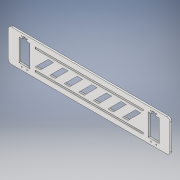
# Autodesk Inventor part: Cuerpo - LateralPrueba
Saved by Autodesk Inventor 2019 (Build 230136000, 136)
## iProperties
Created: 2020-02-14
Part Number: Cuerpo - LateralPrueba
Material: ABS Plastic
Document SubType Name: Modeling
Designer: Mafer1
Density: 1.06 g/cm^3
Appearance: Smooth - White
Mass: 36.6909 g
Surface Area: 287.559 cm^2
Volume: 34.614 cm^3
base_servo: 20.000 mm
altura_servo: 40.000 mm
agujero_servo: 2.000 mm
distancia_agujero_servo: 4.750 mm
soporte: 60.000 mm
largo_base: 200.000 mm
d199: 2.000 mm
d201: 20.000 mm
Author: Mafer1
Autodesk Inventor part; units mm, degrees
ref_plane "YZ Plane" through (0, 0, 0) normal (1, 0, 0) x (0, 1, 0)
ref_plane "XZ Plane" through (0, 0, 0) normal (0, 1, 0) x (-1, 0, 0)
ref_plane "XY Plane" through (0, 0, 0) normal (0, 0, 1) x (1, 0, 0)
sketch "Sketch7" plane through (0, 0, 0) normal (0, 0, 1) x (1, 0, 0)
  line L0 (0, 0) -> (300, 0)
  line L1 (300, 0) -> (300, 60)
  line L2 (300, 60) -> (0, 60)
  line L3 (0, 60) -> (0, 0)
  line L4 (50, 13) -> (250, 13)
  line L5 (250, 13) -> (250, 10)
  line L6 (250, 10) -> (50, 10)
  line L7 (50, 10) -> (50, 13)
  line L8 (150, 13) -> (150, 10) construction
  line L9 (20, 50.8) -> (40.3, 50.8)
  line L10 (40.3, 50.8) -> (40.3, 10)
  line L11 (40.3, 10) -> (20, 10)
  line L12 (20, 10) -> (20, 50.8)
  line L13 (259.7, 50.8) -> (280, 50.8)
  line L14 (280, 50.8) -> (280, 10)
  line L15 (280, 10) -> (259.7, 10)
  line L16 (259.7, 10) -> (259.7, 50.8)
  line L17 (50, 47) -> (250, 47)
  line L18 (250, 47) -> (250, 50)
  line L19 (250, 50) -> (50, 50)
  line L20 (50, 50) -> (50, 47)
  point P0 (50, 48.5)
  point P1 (50, 11.5)
  dimension "d152" = 300
  dimension "d153" = 60
  dimension "d154" = 200
  dimension "d158" = 150
  dimension "d159" = 3
  dimension "d160" = 10
  dimension "d161" = 40.8
  dimension "d162" = 20.3
  dimension "d163" = 20
  dimension "d164" = 20
  dimension "d165" = 10
  dimension "d166" = 10
  dimension "d168" = 10
  constraints: 42 end point, 10 parallel, 5 horizontal, 5 perpendicular, 4 equal length, 4 midpoint, 1 vertical alignment
  measures "d152" distance of L0.start L0.end
  measures "d153" distance of L0.end L1.end
  measures "d154" distance of L4.start L4.end
  measures "d158" distance between parallel lines of L1 L8
  measures "d159" distance between parallel lines of L6 L4
  measures "d160" distance between parallel lines of L0 L6
  measures "d161" distance of L9.end L10.end
  measures "d162" distance of L9.start L9.end
  measures "d163" distance between parallel lines of L12 L3
  measures "d164" distance between parallel lines of L14 L1
  measures "d165" distance between parallel lines of L11 L0
  measures "d166" distance between parallel lines of L0 L15
  measures "d168" distance between parallel lines of L19 L2
extrude "Extrusion7" add sketch "Sketch7" along normal blind 3.3
fillet "Fillet1" radius 6 4 edges at (0, 60, 1.65) (0, 0, 1.65) (300, 60, 1.65) (300, 0, 1.65)
sketch "Sketch9" plane through (0, 0, 3.3) normal (0, 0, 1) x (1, 0, 0)
  arc A0 (294, 0) -> (300, 6) centre (294, 6) ccw projected
  line L0 (300, 6) -> (300, 54) projected
  arc A1 (300, 54) -> (294, 60) centre (294, 54) ccw projected
  line L1 (294, 60) -> (6, 60) projected
  arc A2 (6, 60) -> (0, 54) centre (6, 54) ccw projected
  line L2 (0, 54) -> (0, 6) projected
  arc A3 (0, 6) -> (6, 0) centre (6, 6) ccw projected
  line L3 (6, 0) -> (294, 0) projected
  line L4 (280, 50.8) -> (280, 10) projected
  line L5 (280, 10) -> (259.7, 10) projected
  line L6 (259.7, 10) -> (259.7, 50.8) projected
  line L7 (259.7, 50.8) -> (280, 50.8) projected
  line L8 (40.3, 50.8) -> (40.3, 10) projected
  line L9 (40.3, 10) -> (20, 10) projected
  line L10 (20, 10) -> (20, 50.8) projected
  line L11 (20, 50.8) -> (40.3, 50.8) projected
  line L12 (50, 47) -> (50, 50) projected
  line L13 (50, 50) -> (250, 50) projected
  line L14 (250, 50) -> (250, 47) projected
  line L15 (250, 47) -> (50, 47) projected
  line L16 (250, 13) -> (250, 10) projected
  line L17 (250, 10) -> (50, 10) projected
  line L18 (50, 10) -> (50, 13) projected
  line L19 (50, 13) -> (250, 13) projected
  line L20 (50, 18) -> (74, 42)
  line L21 (74, 42) -> (84, 42)
  line L22 (84, 42) -> (60, 18)
  line L23 (60, 18) -> (50, 18)
  point P0 (0, 0)
  dimension "d172" = 45
  dimension "d173" = 10
  dimension "d175" = 5
  dimension "d182" = 5
  constraints: 8 end point, 2 parallel, 1 horizontal, 1 vertical alignment
  measures "d172" angle of L23 L22
  measures "d173" distance of L20.end L21.end
  measures "d175" distance between parallel lines of L15 L21
  measures "d182" distance between parallel lines of L23 L19
extrude "Extrusion8" cut sketch "Sketch9" against normal blind 3.3 contours L20 L21 L22 L23
pattern_linear "Rectangular Pattern1" count 7 spacing 27 along (1, 0, 0) of "Extrusion8"
sketch "Sketch10" plane through (0, 0, 3.3) normal (0, 0, 1) x (1, 0, 0)
  line L0 (20, 10) -> (20, 50.8) projected
  line L1 (20, 50.8) -> (40.3, 50.8) projected
  line L2 (40.3, 50.8) -> (40.3, 10) projected
  line L3 (40.3, 10) -> (20, 10) projected
  circle A0 centre (25, 54.75) radius 1
  circle A1 centre (35, 54.75) radius 1
  circle A2 centre (25, 5.25) radius 1
  circle A3 centre (35, 5.25) radius 1
  line L4 (259.7, 10) -> (259.7, 50.8) projected
  line L5 (280, 50.8) -> (280, 10) projected
  line L6 (259.7, 50.8) -> (280, 50.8) projected
  line L7 (280, 10) -> (259.7, 10) projected
  circle A4 centre (264.7, 54.75) radius 1
  circle A5 centre (274.7, 54.75) radius 1
  circle A6 centre (264.7, 5.25) radius 1
  circle A7 centre (274.7, 5.25) radius 1
  point P0 (0, 0)
  dimension "d183" = 2
  dimension "d184" = 5
  dimension "d185" = 10
  dimension "d186" = 5
  dimension "d187" = 10
  dimension "d188" = 3.95
  dimension "d189" = 4.75
  dimension "d192" = 2
  dimension "d194" = 10
  dimension "d196" = 10
  dimension "d202" = 5
  constraints: 8 centre point, 6 equal radius, 6 horizontal alignment, 1 vertical alignment
  measures "d183" diameter of A0
  measures "d184" distance from line of L0 A0.centre
  measures "d185" distance of A1.centre A0.centre
  measures "d186" distance from line of L0 A2.centre
  measures "d187" distance of A3.centre A2.centre
  measures "d188" distance from line of L1 A0.centre
  measures "d189" distance from line of L3 A2.centre
  measures "d192" diameter of A4
  measures "d194" distance of A5.centre A4.centre
  measures "d196" distance of A7.centre A6.centre
  measures "d202" distance from line of L4 A4.centre
extrude "Extrusion9" cut sketch "Sketch10" against normal blind 10 contours A0 | A1 | A2 | A3 | A4 | A5 | A6 | A7
sketch "Sketch11" plane through (0, 0, 3.3) normal (0, 0, 1) x (1, 0, 0)
  line L0 (20, 50.8) -> (40.3, 50.8) projected
  line L1 (26.4, 55.9) -> (33.6, 55.9) construction
  line L2 (33.6, 55.9) -> (33.6, 50.8) construction
  line L3 (33.6, 50.8) -> (26.4, 50.8)
  line L4 (26.4, 50.8) -> (26.4, 55.9) construction
  line L5 (20, 10) -> (20, 50.8) projected
  line L6 (40.3, 50.8) -> (40.3, 10) projected
  line L7 (259.7, 50.8) -> (280, 50.8) projected
  line L8 (259.7, 10) -> (259.7, 50.8) projected
  line L9 (26.4, 53.3) -> (28.2205, 55.9)
  line L10 (31.7795, 55.9) -> (33.6, 53.3)
  line L11 (26.4, 50.8) -> (26.4, 53.3)
  line L12 (28.2205, 55.9) -> (31.7795, 55.9)
  line L13 (33.6, 53.3) -> (33.6, 50.8)
  line L14 (266.1, 55.9) -> (273.3, 55.9) construction
  line L15 (273.3, 55.9) -> (273.3, 50.8) construction
  line L16 (273.3, 50.8) -> (266.1, 50.8)
  line L17 (266.1, 50.8) -> (266.1, 55.9) construction
  line L18 (266.1, 53.3) -> (267.9205, 55.9)
  line L19 (271.4795, 55.9) -> (273.3, 53.3)
  line L20 (266.1, 50.8) -> (266.1, 53.3)
  line L21 (267.9205, 55.9) -> (271.4795, 55.9)
  line L22 (273.3, 53.3) -> (273.3, 50.8)
  point P0 (0, 0)
  dimension "d203" = 6.4
  dimension "d205" = 5.1
  dimension "d206" = 7.2
  dimension "d215" = 35
  dimension "d216" = 2.5
  dimension "d217" = 35
  dimension "d219" = 7.2
  dimension "d220" = 35
  dimension "d221" = 35
  dimension "d222" = 6.4
  constraints: 36 end point, 9 point on line, 5 collinear, 4 equal length, 4 horizontal, 4 parallel, 2 perpendicular
  measures "d203" distance between parallel lines of L5 L4
  measures "d205" distance between parallel lines of L0 L1
  measures "d206" distance of L1.start L1.end
  measures "d215" angle of L4 L9
  measures "d216" distance from line of L0 L9.start
  measures "d217" angle of L2 L10
  measures "d219" distance of L14.start L15.start
  measures "d220" angle of L17 L18
  measures "d221" angle of L15 L19
  measures "d222" distance between parallel lines of L8 L17
extrude "Extrusion10" cut sketch "Sketch11" against normal blind 10
equation "\"soporte\" = 60"
equation "\"largo_base\" = 200"
body "Solid2"
